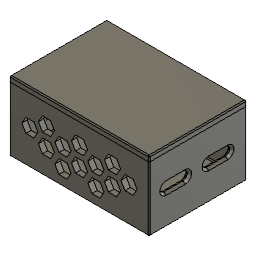
Garage Door Opener C3 Fusion (Autodesk Fusion 360 design; units mm, degrees)
Autodesk Fusion 360 part; units mm, degrees
sketch "Base" plane through (0, 0, 0) normal (0, 1, 0) x (1, 0, 0)
  line L0 (-30, 20) -> (30, 20) construction
  line L1 (30, 20) -> (30, -20) construction
  line L2 (30, -20) -> (-30, -20) construction
  line L3 (-30, -20) -> (-30, 20) construction
  line L4 (-30, 20) -> (30, -20) construction
  line L5 (30, 20) -> (-30, -20) construction
  line L6 (-30.5, 20.5) -> (30.5, 20.5)
  line L7 (30.5, 20.5) -> (30.5, -20.5)
  line L8 (30.5, -20.5) -> (-30.5, -20.5)
  line L9 (-30.5, -20.5) -> (-30.5, 20.5)
  line L10 (-30.5, 20.5) -> (30.5, -20.5) construction
  line L11 (30.5, 20.5) -> (-30.5, -20.5) construction
  line L12 (-33, 23) -> (33, 23)
  line L13 (33, 23) -> (33, -23)
  line L14 (33, -23) -> (-33, -23)
  line L15 (-33, -23) -> (-33, 23)
  line L16 (-33, 23) -> (33, -23) construction
  line L17 (33, 23) -> (-33, -23) construction
  dimension "d3" = 40
  dimension "d4" = 60
  dimension "d5" = 0.5
  dimension "d6" = 0.5
  dimension "d7" = 2.5
  dimension "d8" = 2.5
  constraint horizontal L0
  constraint perpendicular L0 L1
  constraint parallel L0 L2
  constraint parallel L1 L3
  constraint coincident L4 origin
  constraint coincident L5 origin
  constraint horizontal L6
  constraint perpendicular L6 L7
  constraint parallel L6 L8
  constraint parallel L7 L9
  constraint coincident L10 origin
  constraint coincident L11 origin
  constraint horizontal L12
  constraint perpendicular L12 L13
  constraint parallel L12 L14
  constraint parallel L13 L15
  constraint coincident L16 origin
  constraint coincident L17 origin
  measures "d3" distance of L0.start L2.end
  measures "d4" distance of L0.start L0.end
  measures "d5" distance of L0 L6
  measures "d6" distance of L3 L9
  measures "d7" distance of L6 L12
  measures "d8" distance of L9 L15
extrude "Box" add sketch "Base" along normal blind 30.5 contours L6 L7 L8 L9 | L12 L13 L14 L15 makes body 1
shell "Shell1" thickness 2.5 removed faces 1 at (11, 30.5, -7.6667) on bodies 1
sketch "Standoffs" plane through (0, 2.5, 0) normal (0, 1, 0) x (-1, 0, 0)
  line L0 (30.5, 20.5) -> (-30.5, 20.5)
  line L1 (-30.5, 20.5) -> (-30.5, -20.5)
  line L2 (-30.5, -20.5) -> (30.5, -20.5)
  line L3 (30.5, -20.5) -> (30.5, 20.5)
  circle A0 centre (28.5, -18.5) radius 2.875
  line L4 (30.5, 20.5) -> (30.5, -20.5)
  line L5 (30.5, -20.5) -> (-30.5, -20.5)
  circle A1 centre (28.5, -18.5) radius 0.5
  line L6 (30, -20) -> (-30, -20)
  line L7 (30, 20) -> (30, -20)
  dimension "d16" = 5.75
  dimension "d19" = 1
  dimension "d30" = 1.5
  dimension "d31" = 1.5
  constraint concentric A0 A1
  measures "d16" diameter of A0
  measures "d19" diameter of A1
  measures "d30" distance of A0.centre L6
  measures "d31" distance of A0.centre L7
extrude "Extrude2" add sketch "Standoffs" along normal blind 4.5 contours L2 L3 A0 L4 L5 | L2 L3 A0 L4 L5 L6 L7 | A0 L6 L7 | A1 bodies 1
extrude "Extrude4" cut sketch "Standoffs" along normal up to surface (4.5 mm away) contours A1 bodies 1
pattern_linear "R-Pattern1" count 2 spacing 57 along (1, 0, 0) count 2 spacing 37 along (0, 0, 1) of "Extrude2"
sketch "Retainer" plane through (30.5, 0, 0) normal (-1, 0, 0) x (0, 0, 1)
  line L0 (20.5, 7) -> (20.5, 30.5)
  line L1 (-20.5, 30.5) -> (-20.5, 7)
  line L2 (8, 8.6) -> (-8, 8.6)
  line L3 (-8, 8.6) -> (-8, 11.6)
  line L4 (-8, 11.6) -> (8, 11.6)
  line L5 (8, 11.6) -> (8, 8.6)
  line L6 (8, 8.6) -> (-8, 11.6) construction
  line L7 (-8, 8.6) -> (8, 11.6) construction
  line L8 (20.5, 2.5) -> (-20.5, 2.5)
  line L9 (-16.4347, 2.5) -> (16.4347, 2.5)
  line L10 (0, 8.6) -> (0, 2.5) construction
  point P0 (0, 10.1)
  dimension "d32" = 16
  dimension "d33" = 3
  dimension "d34" = 6.1
  constraint horizontal L2
  constraint perpendicular L2 L3
  constraint parallel L2 L4
  constraint parallel L3 L5
  constraint coincident L6 P0
  constraint coincident L7 P0
  constraint midpoint L2 L10.start
  constraint midpoint L9 L10.end
  constraint perpendicular L9 L10
  measures "d32" distance of L3.end L4.end
  measures "d33" distance of L2.end L3.end
  measures "d34" distance of L2 L8
extrude "Retainer" add sketch "Retainer" along normal blind 2.5 draft -45 bodies 1
mirror "Mirror1" about plane through (0, 0, 0) normal (1, 0, 0) of "Retainer"
sketch "PowerSlot" plane through (-33, 0, 0) normal (-1, 0, 0) x (0, 0, 1)
  line L0 (-23, 0) -> (23, 0)
  line L1 (23, 0) -> (23, 30.5)
  line L2 (23, 30.5) -> (-23, 30.5)
  line L3 (-23, 30.5) -> (-23, 0)
  line L4 (-17, 12.7367) -> (-12.5, 12.7367)
  arc A0 (-12.5, 12.7367) -> (-12.5, 16.2367) centre (-12.5, 14.4867) ccw
  line L5 (-12.5, 16.2367) -> (-17, 16.2367)
  arc A1 (-17, 16.2367) -> (-17, 12.7367) centre (-17, 14.4867) ccw
  line L6 (-18.75, 14.4867) -> (-10.75, 14.4867) construction
  line L7 (16.4347, 2.5) -> (-16.4347, 2.5)
  line L8 (-20.5, 7) -> (-20.5, 30.5)
  dimension "d41" = 3.5
  dimension "d48" = 3.5
  dimension "d49" = 12
  dimension "d50" = 4.5
  constraint tangent L4 A0
  constraint tangent A0 L5
  constraint parallel L4 L5
  constraint tangent L5 A1
  constraint tangent L4 A1
  constraint coincident A1 L6.start
  constraint coincident A0 L6.end
  constraint coincident A0.centre L6
  constraint coincident A1.centre L6
  constraint horizontal L6
  measures "d41" diameter of A0
  measures "d48" distance of A1.centre L8
  measures "d49" distance of A1.centre L7.end
  measures "d50" distance of A1.centre A0.centre
sketch "Switchslot" plane through (33, 0, 0) normal (1, 0, 0) x (0, 0, -1)
  line L0 (-23, 0) -> (23, 0)
  line L1 (23, 0) -> (23, 30.5)
  line L2 (23, 30.5) -> (-23, 30.5)
  line L3 (-23, 30.5) -> (-23, 0)
  line L4 (-15, 14) -> (-6, 14)
  arc A0 (-6, 14) -> (-6, 18) centre (-6, 16) ccw
  line L5 (-6, 18) -> (-15, 18)
  arc A1 (-15, 18) -> (-15, 14) centre (-15, 16) ccw
  line L6 (-17, 16) -> (-4, 16) construction
  line L7 (-23, 0) -> (23, 0)
  line L8 (-23, 0) -> (-23, 30.5)
  line L9 (23, 30.5) -> (-23, 30.5)
  line L10 (23, 0) -> (23, 30.5)
  dimension "d46" = 4
  dimension "d51" = 9
  dimension "d122" = 6
  dimension "d125" = 14
  constraint tangent L4 A0
  constraint tangent A0 L5
  constraint parallel L4 L5
  constraint tangent L5 A1
  constraint tangent L4 A1
  constraint coincident A1 L6.start
  constraint coincident A0 L6.end
  constraint coincident A0.centre L6
  constraint coincident A1.centre L6
  constraint perpendicular L1 L6
  measures "d46" diameter of A0
  measures "d51" distance of A1.centre A0.centre
  measures "d122" distance of L6.start L8
  measures "d125" distance of L4 L7
sketch "ledge" plane through (0, 30.5, 0) normal (0, 1, 0) x (-1, 0, 0)
  line L0 (30.5, 20.5) -> (30.5, -20.5)
  line L1 (30.5, -20.5) -> (-30.5, -20.5)
  line L2 (-30.5, -20.5) -> (-30.5, 20.5)
  line L3 (-30.5, 20.5) -> (30.5, 20.5)
  line L4 (33, 23) -> (-33, 23)
  line L5 (-33, 23) -> (-33, -23)
  line L6 (-33, -23) -> (33, -23)
  line L7 (33, -23) -> (33, 23)
  line L8 (31.75, -21.75) -> (-31.75, -21.75)
  line L9 (-31.75, -21.75) -> (-31.75, 21.75)
  line L10 (-31.75, 21.75) -> (31.75, 21.75)
  line L11 (31.75, 21.75) -> (31.75, -21.75)
  line L12 (31.75, -21.75) -> (-31.75, 21.75) construction
  line L13 (-31.75, -21.75) -> (31.75, 21.75) construction
  dimension "d62" = 1.25
  dimension "d64" = 1.25
  constraint horizontal L8
  constraint perpendicular L8 L9
  constraint parallel L8 L10
  constraint parallel L9 L11
  constraint coincident L12 origin
  constraint coincident L13 origin
  measures "d62" distance of L6 L8
  measures "d64" distance of L7 L11
extrude "Extrude9" cut sketch "ledge" against normal blind 3 contours L8 L9 L10 L11 bodies 1
sketch "LidClip" plane through (31.75, 0, 0) normal (-1, 0, 0) x (0, 0, 1)
  line L0 (21.75, 30.5) -> (-21.75, 30.5)
  line L1 (-21.75, 30.5) -> (-21.75, 27.5)
  line L2 (-21.75, 27.5) -> (21.75, 27.5)
  line L3 (21.75, 27.5) -> (21.75, 30.5)
  line L4 (4.25, 29.75) -> (-4.25, 29.75)
  line L5 (-4.25, 29.75) -> (-4.25, 28.25)
  line L6 (-4.25, 28.25) -> (4.25, 28.25)
  line L7 (4.25, 28.25) -> (4.25, 29.75)
  line L8 (4.25, 29.75) -> (-4.25, 28.25) construction
  line L9 (-4.25, 29.75) -> (4.25, 28.25) construction
  line L10 (0, 30.5) -> (0, 29.75) construction
  point P0 (0, 29)
  dimension "d67" = 8.5
  dimension "d68" = 1.5
  dimension "d69" = 1.5
  constraint horizontal L4
  constraint perpendicular L4 L5
  constraint parallel L4 L6
  constraint parallel L5 L7
  constraint coincident L8 P0
  constraint coincident L9 P0
  constraint midpoint L0 L10.start
  constraint midpoint L4 L10.end
  constraint perpendicular L4 L10
  measures "d67" distance of L5.end L6.end
  measures "d68" distance of L4.end L5.end
  measures "d69" distance of L2 P0
extrude "Lid Retainer" add sketch "LidClip" along normal blind 0.8333 draft -45 contours L4 L5 L6 L7 bodies 1
mirror "Mirror2" about plane through (0, 0, 0) normal (1, 0, 0) of "Lid Retainer"
extrude "Lid" add sketch "ledge" 1 faces at (-10.5833, 30.5, -22.5833) along normal blind 2.5 and the other way blind 3 separate body contours L0 L1 L2 L3 | L8 L9 L10 L11 on bodies 1 makes body 2
shell "Lid shell" thickness 2.5 removed faces 1 at (11, 27.5, -7.6667) on bodies 2
extrude "Extrude12" cut sketch "ledge" against normal up to surface (3 mm away) contours L4 L5 L6 L7 bodies 2
extrude "Extrude13" cut sketch "LidClip" along normal blind 0.8333 draft -45 contours L4 L5 L6 L7 bodies 2
mirror "Mirror3" about plane through (0, 0, 0) normal (1, 0, 0) of "Extrude13"
sketch "Honeycomb" plane through (0, 0, -23) normal (0, 0, -1) x (-1, 0, 0)
  line L0 (33, 30.5) -> (-33, 30.5)
  line L1 (1.7854, 8.7111) -> (3.6854, 12.002)
  line L2 (3.6854, 12.002) -> (1.7854, 15.2929)
  line L3 (1.7854, 15.2929) -> (-2.0146, 15.2929)
  line L4 (-2.0146, 15.2929) -> (-3.9146, 12.002)
  line L5 (-3.9146, 12.002) -> (-2.0146, 8.7111)
  line L6 (-2.0146, 8.7111) -> (1.7854, 8.7111)
  line L7 (-35.4306, 20.7006) -> (35.3521, 20.7006)
  line L8 (35.3521, 20.7006) -> (35.3521, 3.4959)
  line L9 (35.3521, 3.4959) -> (-35.4306, 3.4959)
  line L10 (-35.4306, 3.4959) -> (-35.4306, 20.7006)
  line L11 (-0.1146, 12.002) -> (-2.9646, 13.6474) construction
  line L12 (-0.1146, 12.002) -> (2.7354, 13.6474) construction
  line L13 (-13.8031, 6.2929) -> (-17.6031, 6.2929)
  line L14 (-19.5031, 3.002) -> (-17.6031, -0.2889)
  line L15 (-17.6031, 6.2929) -> (-19.5031, 3.002)
  line L16 (-17.6031, -0.2889) -> (-13.8031, -0.2889)
  line L17 (-13.8031, -0.2889) -> (-11.9031, 3.002)
  line L18 (-11.9031, 3.002) -> (-13.8031, 6.2929)
  line L19 (-21.5973, 10.7929) -> (-25.3973, 10.7929)
  line L20 (-27.2973, 7.502) -> (-25.3973, 4.2111)
  line L21 (-25.3973, 10.7929) -> (-27.2973, 7.502)
  line L22 (-25.3973, 4.2111) -> (-21.5973, 4.2111)
  line L23 (-21.5973, 4.2111) -> (-19.6973, 7.502)
  line L24 (-19.6973, 7.502) -> (-21.5973, 10.7929)
  line L25 (-29.3915, 15.2929) -> (-33.1915, 15.2929)
  line L26 (-35.0915, 12.002) -> (-33.1915, 8.7111)
  line L27 (-33.1915, 15.2929) -> (-35.0915, 12.002)
  line L28 (-33.1915, 8.7111) -> (-29.3915, 8.7111)
  line L29 (-29.3915, 8.7111) -> (-27.4915, 12.002)
  line L30 (-27.4915, 12.002) -> (-29.3915, 15.2929)
  line L31 (1.7854, 6.2929) -> (-2.0146, 6.2929)
  line L32 (-3.9146, 3.002) -> (-2.0146, -0.2889)
  line L33 (-2.0146, 6.2929) -> (-3.9146, 3.002)
  line L34 (-2.0146, -0.2889) -> (1.7854, -0.2889)
  line L35 (1.7854, -0.2889) -> (3.6854, 3.002)
  line L36 (3.6854, 3.002) -> (1.7854, 6.2929)
  line L37 (-6.0088, 10.7929) -> (-9.8088, 10.7929)
  line L38 (-11.7088, 7.502) -> (-9.8088, 4.2111)
  line L39 (-9.8088, 10.7929) -> (-11.7088, 7.502)
  line L40 (-9.8088, 4.2111) -> (-6.0088, 4.2111)
  line L41 (-6.0088, 4.2111) -> (-4.1088, 7.502)
  line L42 (-4.1088, 7.502) -> (-6.0088, 10.7929)
  line L43 (-13.8031, 15.2929) -> (-17.6031, 15.2929)
  line L44 (-19.5031, 12.002) -> (-17.6031, 8.7111)
  line L45 (-17.6031, 15.2929) -> (-19.5031, 12.002)
  line L46 (-17.6031, 8.7111) -> (-13.8031, 8.7111)
  line L47 (-13.8031, 8.7111) -> (-11.9031, 12.002)
  line L48 (-11.9031, 12.002) -> (-13.8031, 15.2929)
  line L49 (-21.5973, 19.7929) -> (-25.3973, 19.7929)
  line L50 (-27.2973, 16.502) -> (-25.3973, 13.2111)
  line L51 (-25.3973, 19.7929) -> (-27.2973, 16.502)
  line L52 (-25.3973, 13.2111) -> (-21.5973, 13.2111)
  line L53 (-21.5973, 13.2111) -> (-19.6973, 16.502)
  line L54 (-19.6973, 16.502) -> (-21.5973, 19.7929)
  line L55 (-29.3915, 24.2929) -> (-33.1915, 24.2929)
  line L56 (-35.0915, 21.002) -> (-33.1915, 17.7111)
  line L57 (-33.1915, 24.2929) -> (-35.0915, 21.002)
  line L58 (-33.1915, 17.7111) -> (-29.3915, 17.7111)
  line L59 (-29.3915, 17.7111) -> (-27.4915, 21.002)
  line L60 (-27.4915, 21.002) -> (-29.3915, 24.2929)
  line L61 (17.3738, 6.2929) -> (13.5738, 6.2929)
  line L62 (11.6738, 3.002) -> (13.5738, -0.2889)
  line L63 (13.5738, 6.2929) -> (11.6738, 3.002)
  line L64 (13.5738, -0.2889) -> (17.3738, -0.2889)
  line L65 (17.3738, -0.2889) -> (19.2738, 3.002)
  line L66 (19.2738, 3.002) -> (17.3738, 6.2929)
  line L67 (9.5796, 10.7929) -> (5.7796, 10.7929)
  line L68 (3.8796, 7.502) -> (5.7796, 4.2111)
  line L69 (5.7796, 10.7929) -> (3.8796, 7.502)
  line L70 (5.7796, 4.2111) -> (9.5796, 4.2111)
  line L71 (9.5796, 4.2111) -> (11.4796, 7.502)
  line L72 (11.4796, 7.502) -> (9.5796, 10.7929)
  line L73 (-6.0088, 19.7929) -> (-9.8088, 19.7929)
  line L74 (-11.7088, 16.502) -> (-9.8088, 13.2111)
  line L75 (-9.8088, 19.7929) -> (-11.7088, 16.502)
  line L76 (-9.8088, 13.2111) -> (-6.0088, 13.2111)
  line L77 (-6.0088, 13.2111) -> (-4.1088, 16.502)
  line L78 (-4.1088, 16.502) -> (-6.0088, 19.7929)
  line L79 (-13.8031, 24.2929) -> (-17.6031, 24.2929)
  line L80 (-19.5031, 21.002) -> (-17.6031, 17.7111)
  line L81 (-17.6031, 24.2929) -> (-19.5031, 21.002)
  line L82 (-17.6031, 17.7111) -> (-13.8031, 17.7111)
  line L83 (-13.8031, 17.7111) -> (-11.9031, 21.002)
  line L84 (-11.9031, 21.002) -> (-13.8031, 24.2929)
  line L85 (25.1681, 10.7929) -> (21.3681, 10.7929)
  line L86 (19.4681, 7.502) -> (21.3681, 4.2111)
  line L87 (21.3681, 10.7929) -> (19.4681, 7.502)
  line L88 (21.3681, 4.2111) -> (25.1681, 4.2111)
  line L89 (25.1681, 4.2111) -> (27.0681, 7.502)
  line L90 (27.0681, 7.502) -> (25.1681, 10.7929)
  line L91 (17.3738, 15.2929) -> (13.5738, 15.2929)
  line L92 (11.6738, 12.002) -> (13.5738, 8.7111)
  line L93 (13.5738, 15.2929) -> (11.6738, 12.002)
  line L94 (13.5738, 8.7111) -> (17.3738, 8.7111)
  line L95 (17.3738, 8.7111) -> (19.2738, 12.002)
  line L96 (19.2738, 12.002) -> (17.3738, 15.2929)
  line L97 (9.5796, 19.7929) -> (5.7796, 19.7929)
  line L98 (3.8796, 16.502) -> (5.7796, 13.2111)
  line L99 (5.7796, 19.7929) -> (3.8796, 16.502)
  line L100 (5.7796, 13.2111) -> (9.5796, 13.2111)
  line L101 (9.5796, 13.2111) -> (11.4796, 16.502)
  line L102 (11.4796, 16.502) -> (9.5796, 19.7929)
  line L103 (1.7854, 24.2929) -> (-2.0146, 24.2929)
  line L104 (-3.9146, 21.002) -> (-2.0146, 17.7111)
  line L105 (-2.0146, 24.2929) -> (-3.9146, 21.002)
  line L106 (-2.0146, 17.7111) -> (1.7854, 17.7111)
  line L107 (1.7854, 17.7111) -> (3.6854, 21.002)
  line L108 (3.6854, 21.002) -> (1.7854, 24.2929)
  line L109 (32.9623, 15.2929) -> (29.1623, 15.2929)
  line L110 (27.2623, 12.002) -> (29.1623, 8.7111)
  line L111 (29.1623, 15.2929) -> (27.2623, 12.002)
  line L112 (29.1623, 8.7111) -> (32.9623, 8.7111)
  line L113 (32.9623, 8.7111) -> (34.8623, 12.002)
  line L114 (34.8623, 12.002) -> (32.9623, 15.2929)
  line L115 (25.1681, 19.7929) -> (21.3681, 19.7929)
  line L116 (19.4681, 16.502) -> (21.3681, 13.2111)
  line L117 (21.3681, 19.7929) -> (19.4681, 16.502)
  line L118 (21.3681, 13.2111) -> (25.1681, 13.2111)
  line L119 (25.1681, 13.2111) -> (27.0681, 16.502)
  line L120 (27.0681, 16.502) -> (25.1681, 19.7929)
  line L121 (17.3738, 24.2929) -> (13.5738, 24.2929)
  line L122 (11.6738, 21.002) -> (13.5738, 17.7111)
  line L123 (13.5738, 24.2929) -> (11.6738, 21.002)
  line L124 (13.5738, 17.7111) -> (17.3738, 17.7111)
  line L125 (17.3738, 17.7111) -> (19.2738, 21.002)
  line L126 (19.2738, 21.002) -> (17.3738, 24.2929)
  line L127 (32.9623, 24.2929) -> (29.1623, 24.2929)
  line L128 (27.2623, 21.002) -> (29.1623, 17.7111)
  line L129 (29.1623, 24.2929) -> (27.2623, 21.002)
  line L130 (29.1623, 17.7111) -> (32.9623, 17.7111)
  line L131 (32.9623, 17.7111) -> (34.8623, 21.002)
  line L132 (34.8623, 21.002) -> (32.9623, 24.2929)
  line L133 (-33, 0) -> (33, 0)
  line L134 (33, 0) -> (33, 30.5)
  line L135 (-33, 30.5) -> (-33, 0)
  point P0 (-0.1146, 12.002)
  dimension "d105" = 3.8
  dimension "d108" = 9
  dimension "d109" = 9
  constraint horizontal L6
  constraint horizontal L7
  constraint vertical L8
  constraint horizontal L9
  constraint vertical L10
  constraint coincident P0 L11.start
  constraint midpoint L4 L11.end
  constraint midpoint L2 L12.end
  measures "d105" distance of L1.start P0
extrude "Extrude17" cut sketch "PowerSlot" against normal up to surface (2.5 mm away) contours L4 A0 L5 A1 bodies 1
extrude "Extrude18" cut sketch "Switchslot" against normal up to surface (2.5 mm away) contours L4 A0 L5 A1 bodies 1
extrude "Extrude19" cut sketch "Honeycomb" against normal up to surface (46 mm away) contours L7 L122 L124 L125 | L7 L121 L122 L123 L125 L126 | L7 L79 L80 L81 L83 L84 | L7 L80 L82 L83 | L7 L104 L106 L107 | L7 L103 L104 L105 L107 L108 | L1 L2 L3 L4 L5 L6 | L37 L38 L39 L40 L41 L42 | L43 L44 L45 L46 L47 L48 | L49 L50 L51 L52 L53 L54 | L67 L68 L69 L70 L71 L72 | L73 L74 L75 L76 L77 L78 | L91 L92 L93 L94 L95 L96 | L97 L98 L99 L100 L101 L102 | L115 L116 L117 L118 L119 L120 bodies 1
fillet "Fillet7" radius 0.5 8 edges at (33, 15.25, -23) (33, 0, 0) (0, 0, -23) (33, 15.25, 23) (0, 0, 23) (-33, 0, 0) (-33, 15.25, -23) (-33, 15.25, 23) on bodies 1
chamfer "Chamfer6" distance 0.5 angle 45 4 edges at (0, 2.5, 20.5) (-30.5, 2.5, 0) (30.5, 2.5, 0) (0, 2.5, -20.5) on bodies 1
chamfer "Chamfer6" distance 0.5 angle 45 4 edges at (-26.4671, 2.5, -16.4671) (-26.4671, 2.5, 16.4671) (26.4671, 2.5, 16.4671) (26.4671, 2.5, -16.4671) on bodies 1
chamfer "Chamfer8" distance 1 angle 45 8 edges at (30.5, 14, 10.5) (30.5, 16, 4) (30.5, 18, 10.5) (30.5, 16, 17) (33, 14, 10.5) (33, 16, 17) (33, 18, 10.5) (33, 16, 4) on bodies 1
chamfer "Chamfer8" distance 1 angle 45 8 edges at (-33, 12.7367, -14.75) (-33, 14.4867, -18.75) (-33, 16.2367, -14.75) (-33, 14.4867, -10.75) (-30.5, 12.7367, -14.75) (-30.5, 14.4867, -10.75) (-30.5, 16.2367, -14.75) (-30.5, 14.4867, -18.75) on bodies 1
chamfer "Chamfer9" distance 0.5 angle 45 8 edges at (-33, 33, 0) (0, 33, -23) (0, 33, 23) (33, 33, 0) (33, 31.75, 23) (-33, 31.75, 23) (-33, 31.75, -23) (33, 31.75, -23) on bodies 2
pattern_linear "R-Pattern2" count 2 spacing 20 along (0, 0, -1) of "Extrude18", "Chamfer8"
equation "skin = 2.5 mm"
equation "fit = 0.5 mm"
equation "d5 = fit"
equation "d6 = fit"
equation "d7 = skin"
equation "d8 = skin"
equation "d13 = 28 mm + skin"
equation "d15 = skin"
equation "d16 = 4 mm + fit + ( skin / 2 )"
equation "d20 = standoff"
equation "d28 = 60 mm - 3 mm"
equation "d29 = 40 mm - 3 mm"
equation "d34 = standoff + pcb_tickness"
equation "d35 = 2 mm + fit"
equation "standoff = 4.5 mm"
equation "pcb_tickness = 1.6 mm"
equation "lip = 3 mm"
equation "d62 = skin / 2"
equation "d64 = skin / 2"
equation "d65 = -lip"
equation "d69 = lip / 2"
equation "d70 = skin / 3"
equation "d74 = skin"
equation "d76 = lip"
equation "d78 = skin"
equation "d81 = skin / 3"
named bodies: "Shell", "Lid"
